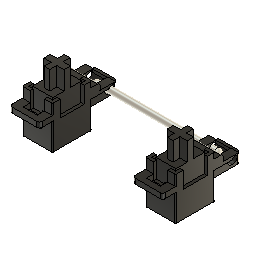
Choc v2 Stabilizer v8 (Autodesk Fusion 360 design; units mm, degrees)
Autodesk Fusion 360 part; units mm, degrees
note: some values were not read from the file. Chosen so that the rebuilt part matches the saved one: which bodies a step acts on; a side; which face or edge a step refers to.
ref_plane "WorkPlane1" through (0, 0, -5.4) normal (0, 0, 1) x (1, 0, 0)
ref_plane "Ext Bottom" through (0, 0, -2) normal (0, 0, 1) x (1, 0, 0)
ref_plane "WorkPlane3" through (0, 0, -0.2) normal (0, 0, 1) x (1, 0, 0)
sketch "Case Top" plane through (0, 0, 0) normal (0, 0, 1) x (1, 0, 0)
  line L0 (1.3, -2.05) -> (-1.3, -2.05)
  line L1 (-1.3, -2.05) -> (-1.3, 2.05)
  line L2 (-1.3, 2.05) -> (1.3, 2.05)
  line L3 (1.3, 2.05) -> (1.3, -2.05)
  line L4 (1.3, -2.05) -> (-1.3, 2.05) construction
  line L5 (-1.3, -2.05) -> (1.3, 2.05) construction
  line L6 (2.9, -3.8) -> (-2.9, -3.8)
  line L7 (-2.9, -3.8) -> (-2.9, 3.8)
  line L8 (-2.9, 3.8) -> (2.9, 3.8)
  line L9 (2.9, 3.8) -> (2.9, -3.8)
  line L10 (2.9, -3.8) -> (-2.9, 3.8) construction
  line L11 (-2.9, -3.8) -> (2.9, 3.8) construction
  line L12 (-2.9, -3.8) -> (2.9, -3.8)
  line L13 (2.9, -3.8) -> (2.9, -6.3)
  line L14 (2.9, -6.3) -> (-2.9, -6.3)
  line L15 (-2.9, -6.3) -> (-2.9, -3.8)
  line L16 (-2.9, 3.8) -> (2.9, 3.8)
  line L17 (2.9, 3.8) -> (2.9, 9.4)
  line L18 (2.9, 9.4) -> (-2.9, 9.4)
  line L19 (-2.9, 9.4) -> (-2.9, 3.8)
  line L20 (-2.9, 5.4) -> (2.9, 5.4)
  line L21 (-2.9, -2.3) -> (-2.3, -2.3)
  line L22 (-2.3, -2.3) -> (-2.3, -3.2)
  line L23 (-2.3, -3.2) -> (-1.4, -3.2)
  line L24 (-1.4, -3.2) -> (-1.4, -3.8)
  line L25 (0, 2.5) -> (0, 20)
  line L26 (2.9, -2.3) -> (2.3, -2.3)
  line L27 (2.3, -2.3) -> (2.3, -3.2)
  line L28 (2.3, -3.2) -> (1.4, -3.2)
  line L29 (1.4, -3.2) -> (1.4, -3.8)
  line L30 (20, 0) -> (2.5, 0)
  line L31 (-2.9, 2.3) -> (-2.3, 2.3)
  line L32 (-2.3, 2.3) -> (-2.3, 3.2)
  line L33 (-2.3, 3.2) -> (-1.4, 3.2)
  line L34 (-1.4, 3.2) -> (-1.4, 3.8)
  line L35 (1.4, 3.2) -> (1.4, 3.8)
  line L36 (2.3, 3.2) -> (1.4, 3.2)
  line L37 (2.3, 2.3) -> (2.3, 3.2)
  line L38 (2.9, 2.3) -> (2.3, 2.3)
  line L39 (-2.3, 2.3) -> (-2.3, -2.3)
  line L40 (2.3, -2.3) -> (2.3, 2.3)
  line L41 (-1.4, 3.2) -> (1.4, 3.2)
  line L42 (-1.4, -3.2) -> (1.4, -3.2)
  line L43 (2.15, 9.4) -> (2.15, 3.8)
  line L44 (-2.15, 9.4) -> (-2.15, 3.8)
  line L45 (-1, 9.4) -> (1, 9.4)
  line L46 (1, 9.4) -> (1, 9.9)
  line L47 (1, 9.9) -> (-1, 9.9)
  line L48 (-1, 9.9) -> (-1, 9.4)
  line L49 (-2.9, 8.4) -> (2.9, 8.4)
  line L50 (-0.95, -3.8) -> (0.95, -3.8)
  line L51 (0.95, -3.8) -> (0.95, -4.8)
  line L52 (0.95, -4.8) -> (-0.95, -4.8)
  line L53 (-0.95, -4.8) -> (-0.95, -3.8)
  line L54 (1.4, 8.4) -> (1.4, 3.8)
  line L55 (-1.4, 8.4) -> (-1.4, 3.8)
  line L56 (11.7972, 15.6555) -> (-12.0028, 15.6555)
  dimension "d3" = 2.6
  dimension "d4" = 4.1
  dimension "d5" = 7.6
  dimension "d6" = 5.8
  dimension "d7" = 2.5
  dimension "d8" = 5.6
  dimension "d9" = 4
  dimension "d10" = 1.5
  dimension "d11" = 1.5
  dimension "d12" = 0.6
  dimension "d13" = 0.6
  dimension "d14" = 4.3
  dimension "d16" = 2
  dimension "d17" = 0.5
  dimension "d26" = 4.6
  dimension "d36" = 1.9
  dimension "d37" = 1
  dimension "d49" = 2.8
  dimension "ParameterA" = 23.8
  constraint horizontal L0
  constraint perpendicular L0 L1
  constraint parallel L0 L2
  constraint parallel L1 L3
  constraint coincident L4 origin
  constraint coincident L5 origin
  constraint horizontal L6
  constraint perpendicular L6 L7
  constraint parallel L6 L8
  constraint parallel L7 L9
  constraint coincident L10 origin
  constraint coincident L11 origin
  constraint horizontal L12
  constraint vertical L13
  constraint horizontal L14
  constraint vertical L15
  constraint coincident L6.start L9.end
  constraint horizontal L16
  constraint vertical L17
  constraint horizontal L18
  constraint vertical L19
  constraint coincident L8.end L9.start
  constraint coincident L19 L20.start
  constraint coincident L17 L20.end
  constraint perpendicular L17 L20
  constraint coincident L7 L21.start
  constraint perpendicular L7 L21
  constraint perpendicular L21 L22
  constraint perpendicular L22 L23
  constraint coincident L12 L24.end
  constraint vertical L24
  constraint symmetric L21.start L25 L26.start
  constraint symmetric L21.end L25 L26.end
  constraint symmetric L22.end L25 L27.end
  constraint symmetric L23.end L25 L28.end
  constraint symmetric L24.end L25 L29.end
  constraint symmetric L21.start L30 L31.start
  constraint symmetric L21.end L30 L31.end
  constraint symmetric L22.end L30 L32.end
  constraint symmetric L23.end L30 L33.end
  constraint symmetric L24.end L30 L34.end
  constraint symmetric L26.start L30 L38.start
  constraint symmetric L26.end L30 L37.start
  constraint symmetric L27.end L30 L36.start
  constraint symmetric L28.end L30 L35.start
  constraint symmetric L29.end L30 L35.end
  constraint coincident L18 L43.start
  constraint coincident L16 L43.end
  constraint perpendicular L16 L43
  constraint symmetric L25 L43.start L44.start
  constraint symmetric L25 L43.end L44.end
  constraint horizontal L45
  constraint vertical L46
  constraint horizontal L47
  constraint vertical L48
  constraint coincident L18 L45.start
  constraint symmetric L25 L46 L48
  constraint coincident L19 L49.start
  constraint coincident L17 L49.end
  constraint perpendicular L17 L49
  constraint horizontal L50
  constraint vertical L51
  constraint horizontal L52
  constraint vertical L53
  constraint coincident L6 L50.start
  constraint symmetric L25 L51 L53
  constraint coincident L49 L54.start
  constraint coincident L16 L35.end
  constraint vertical L54
  constraint symmetric L25 L54.start L55.start
  constraint symmetric L25 L35.end L34.end
  constraint horizontal L56
  measures "d3" distance of L0.start L0.end
  measures "d4" distance of L0.start L2.end
  measures "d5" distance of L6.start L8.end
  measures "d6" distance of L6.start L6.end
  measures "d7" distance of L6.start L13.end
  measures "d8" distance of L8.end L17.end
  measures "d9" distance of L18 L20
  measures "d10" distance of L7 L24
  measures "d11" distance of L6 L21
  measures "d12" distance of L21.start L21.end
  measures "d13" distance of L23.end L24.end
  measures "d14" distance of L43 L44
  measures "d16" distance of L46.end L47.end
  measures "d17" distance of L45.end L46.end
  measures "d26" distance of L8 L49
  measures "d36" distance of L51.end L52.end
  measures "d37" distance of L50.end L51.end
  measures "d49" distance of L54 L55
  measures "ParameterA" distance of L56.start L56.end
extrude "Extrude1" add sketch "Case Top" against normal up to surface (5.2 mm away) from surface at -0.2 contours L0 L1 L2 L3 | L6 L9 L12 L26 L27 L28 L29 | L6 L12 L24 L29 L42 L50 | L9 L26 L38 L40 | L22 L23 L27 L28 L32 L33 L36 L37 L39 L40 L41 L42 | L6 L7 L12 L21 L22 L23 L24 | L8 L9 L16 L35 L36 L37 L38 | L7 L21 L31 L39 | L8 L16 L25 L35 L41 | L7 L8 L16 L31 L32 L33 L34 | L8 L16 L25 L34 L41 makes body 1
extrude "Extrude2" add sketch "Case Top" along normal blind 3.2 from surface at -0.2 contours L6 L9 L12 L26 L27 L28 L29 | L6 L7 L12 L21 L22 L23 L24 | L8 L9 L16 L35 L36 L37 L38 | L7 L8 L16 L31 L32 L33 L34 bodies 1
extrude "Extrude4" cut sketch "Case Top" against normal up to surface (5.4 mm away) contours L0 L1 L2 L3 bodies 1
extrude "Extrude3" cut sketch "Case Top" against normal up to surface (4.8 mm away) contours L22 L23 L27 L28 L32 L33 L36 L37 L39 L40 L41 L42 bodies 1
extrude "Extrude5" add sketch "Case Top" along normal blind 0.6 separate body contours L8 L16 L17 L20 L43 | L8 L16 L20 L43 L54 | L17 L20 L43 L49 | L8 L16 L20 L25 L54 | L20 L43 L49 L54 | L8 L16 L19 L20 L44 | L8 L16 L20 L25 L55 | L20 L25 L49 L54 | L8 L16 L20 L44 L55 | L19 L20 L44 L49 | L20 L25 L49 L55 | L20 L44 L49 L55 makes body 2
extrude "Extrude6" add sketch "Case Top" along normal blind 1.9 contours L8 L16 L17 L20 L43 | L8 L16 L20 L43 L54 | L8 L16 L20 L25 L54 | L8 L16 L19 L20 L44 | L8 L16 L20 L25 L55 | L8 L16 L20 L44 L55 bodies 1 2
extrude "Extrude7" add sketch "Case Top" against normal up to surface (2 mm away) contours L8 L16 L20 L43 L54 | L8 L16 L20 L25 L54 | L20 L43 L49 L54 | L8 L16 L20 L25 L55 | L20 L25 L49 L54 | L18 L25 L43 L45 L49 | L8 L16 L20 L44 L55 | L20 L25 L49 L55 | L20 L44 L49 L55 | L18 L25 L44 L45 L49 bodies 1
extrude "Extrude8" add sketch "Case Top" against normal blind 1 from surface at -1 contours L18 L25 L45 L46 L47 | L18 L25 L45 L47 L48 bodies 1
extrude "Extrude9" add sketch "Case Top" along normal blind 1 contours L6 L12 L13 L14 L15 L51 L52 L53 bodies 1
extrude "Extrude10" add sketch "Case Top" against normal blind 1.5 from surface at -0.5 contours L6 L12 L50 L51 L52 L53 bodies 1
extrude "Extrude11" cut sketch "Case Top" along normal up to surface (0.6 mm away) and the other way blind 1.4 contours L8 L16 L20 L25 L54 | L8 L16 L20 L25 L55 | L20 L25 L49 L54 | L20 L25 L49 L55 bodies 1
fillet "Fillet1" radius 0.2 16 edges at (-2.9, 3.8, -2.7) (0, 3.8, -5.4) (2.9, 3.8, -2.7) (-2.9, 3.8, 2.45) (-2.9, -3.8, 2) (-2.9, -3.8, -2.7) (-2.9, 0, -5.4) (2.9, 0, -5.4) (0, -3.8, -5.4) (2.9, -3.8, -2.7) (2.9, -3.8, 2) (2.9, 3.8, 2.45) (1.3, -2.05, -5.1) (1.3, 2.05, -5.1) (-1.3, 2.05, -5.1) (-1.3, -2.05, -5.1) on bodies 1
fillet "Fillet2" radius 0.5 5 edges at (0, 5.4, 1.9) (-2.15, 9.4, -1) (2.15, 9.4, -1) (-2.9, -6.3, 0.5) (2.9, -6.3, 0.5) on bodies 1
chamfer "Chamfer1" distance 0.7 angle 45 2 edges at (0, -4.8, -0.5) (0, -4.8, -2) on bodies 1
chamfer "Chamfer2" distance 0.5 angle 45 1 edges at (0, 9.9, -2) on bodies 1
move_face "OffsetFaces1" offset -0.4 3 faces at (0.3167, -4.8, 0.3333) (0.95, -4.1333, 0.3333) (-0.95, -4.4667, 0.3333) on bodies 1
sketch "Case Side2" plane through (-2.15, 0, 0) normal (-1, 0, 0) x (0, -1, 0)
  line L0 (-8.4, -1.4) -> (-3.8, -1.4)
  arc A0 (-8.8655, -0.5741) -> (-8.4, -1.4) centre (-7.9, -0.5741) ccw
  line L1 (-8.8655, -0.5741) -> (-8.8655, 0.3914)
  circle A1 centre (-7.9, -0.8) radius 0.6
  arc A2 (-8.4, -1.4) -> (-7.9, 0.3914) centre (-7.9, -0.5741) ccw
  line L2 (-8.4, 0) -> (-8.4, 0.6)
  line L3 (-7.9, 0.3914) -> (-8.8655, 0.3914)
  line L4 (-7.9, -1.1252) -> (-7.9, 0.2054) construction
  dimension "d55" = 1.2
  dimension "WireYAdjust" = 0.5
  constraint coincident L0.start A0.end
  constraint perpendicular L0 L1
  constraint tangent A0 L1
  constraint tangent L0 A1
  constraint tangent A0 A2
  constraint horizontal L3
  constraint coincident L1.end L3.end
  constraint vertical L4
  constraint coincident A1.centre L4
  constraint coincident A0.centre L4
  constraint tangent A2 L3
  measures "d55" diameter of A1
  measures "WireYAdjust" distance of A1.centre L2
extrude "Extrude12" cut sketch "Case Side2" along normal up to surface (-5.05 mm away) and the other way up to surface (-0.75 mm away) contours A1 | L0 A0 L1 A2 L3 | L0 A2 bodies 1
sketch "Stem Top" plane through (0, 0, -0.2) normal (0, 0, 1) x (1, 0, 0)
  line L0 (-1.95, 2.8) -> (1.95, 2.8)
  line L1 (1.95, 2.8) -> (1.95, -2.8)
  line L2 (1.95, -2.8) -> (-1.95, -2.8)
  line L3 (-1.95, -2.8) -> (-1.95, 2.8)
  line L4 (-1.95, 2.8) -> (1.95, -2.8) construction
  line L5 (1.95, 2.8) -> (-1.95, -2.8) construction
  line L6 (-0.55, -0.615) -> (-1.95, -0.615)
  line L7 (-0.55, -0.615) -> (-0.55, -1.95)
  line L8 (20, 0) -> (2.5, 0)
  line L9 (-0.55, 0.615) -> (-1.95, 0.615)
  line L10 (-0.55, 0.615) -> (-0.55, 1.95)
  line L11 (0, 2.5) -> (0, 20)
  line L12 (0.55, -0.615) -> (1.95, -0.615)
  line L13 (0.55, -0.615) -> (0.55, -1.95)
  line L14 (0.55, 0.615) -> (0.55, 1.95)
  line L15 (0.55, 0.615) -> (1.95, 0.615)
  line L16 (0.55, -1.95) -> (-0.55, -1.95)
  line L17 (0.55, 1.95) -> (-0.55, 1.95)
  dimension "d60" = 3.9
  dimension "d61" = 5.6
  dimension "d62" = 1.23
  dimension "d63" = 1.1
  dimension "d64" = 3.9
  constraint horizontal L0
  constraint perpendicular L0 L1
  constraint parallel L0 L2
  constraint parallel L1 L3
  constraint coincident L4 origin
  constraint coincident L5 origin
  constraint coincident L3 L6.end
  constraint perpendicular L3 L6
  constraint perpendicular L6 L7
  constraint symmetric L6.start L8 L9.start
  constraint symmetric L6.end L8 L9.end
  constraint symmetric L7.end L8 L10.end
  constraint symmetric L6.start L11 L12.start
  constraint symmetric L6.end L11 L12.end
  constraint symmetric L7.end L11 L13.end
  constraint symmetric L9.start L11 L14.start
  constraint symmetric L9.end L11 L15.end
  constraint symmetric L10.end L11 L14.end
  measures "d60" distance of L0.start L0.end
  measures "d61" distance of L0.start L2.end
  measures "d62" distance of L6 L9
  measures "d63" distance of L7 L13
  measures "d64" distance of L16 L17
extrude "Extrude13" add sketch "Stem Top" along normal blind 3.6 separate body contours L1 L3 L6 L7 L9 L10 L12 L13 L14 L15 L16 L17 makes body 3
extrude "Extrude14" add sketch "Stem Top" against normal blind 4.5 bodies 3
move_body "Move2" bodies 3 to x (1, 0, 0) y (0, 1, 0) z (0, 0, 1) at (0, 0, 3.2)
sketch "Fill Hole Top" plane through (0, 0, 0) normal (0, 0, 1) x (1, 0, 0)
  line L0 (3, -4.5) -> (-3, -4.5)
  line L1 (-3, -4.5) -> (-3, 9.4)
  line L2 (-3, 9.4) -> (3, 9.4)
  line L3 (3, 9.4) -> (3, -4.5)
  line L4 (3, -4.5) -> (-3, 9.4) construction
  line L5 (-3, -4.5) -> (3, 9.4) construction
  line L6 (0, 1.75) -> (0, 22.5)
  line L7 (-4, -5.5) -> (-4, 10.4)
  line L8 (-4, 10.4) -> (4, 10.4)
  line L9 (4, 10.4) -> (4, -5.5)
  line L10 (4, -5.5) -> (-4, -5.5)
  line L11 (2.25, 9.4) -> (2.25, 3.9)
  line L12 (2.25, 3.9) -> (3, 3.9)
  line L13 (2.15, 9.4) -> (2.15, 3.8)
  line L14 (-2.9, 3.8) -> (2.9, 3.8)
  line L15 (0, 2.5) -> (0, 20)
  line L16 (-2.25, 3.9) -> (-3, 3.9)
  line L17 (-2.25, 9.4) -> (-2.25, 3.9)
  line L18 (-2.4, -6.3) -> (2.4, -6.3)
  arc A0 (-2.9, -5.8) -> (-2.4, -6.3) centre (-2.4, -5.8) ccw
  line L19 (-2.9, -3.6) -> (-2.9, -5.8)
  arc A1 (2.4, -6.3) -> (2.9, -5.8) centre (2.4, -5.8) ccw
  line L20 (2.9, -5.8) -> (2.9, -3.6)
  line L21 (-3, -3.6) -> (-3, -5.8)
  arc A2 (-3, -5.8) -> (-2.4, -6.4) centre (-2.4, -5.8) ccw
  line L22 (-2.4, -6.4) -> (2.4, -6.4)
  arc A3 (2.4, -6.4) -> (3, -5.8) centre (2.4, -5.8) ccw
  line L23 (3, -5.8) -> (3, -3.6)
  line L24 (-2.25, 3.9) -> (2.25, 3.9)
  point P0 (0, 2.45)
  point P1 (-2.15, 9.4)
  dimension "d72" = 6
  dimension "d74" = -1
  dimension "d76" = 0.1
  dimension "d77" = 0.1
  dimension "d78" = 8.3
  dimension "d85" = 0.1
  constraint horizontal L0
  constraint perpendicular L0 L1
  constraint parallel L0 L2
  constraint parallel L1 L3
  constraint coincident L4 P0
  constraint coincident L5 P0
  constraint coincident P0 L6
  constraint coincident L2 P1
  constraint coincident L2 L11.start
  constraint perpendicular L2 L11
  constraint coincident L3 L12.end
  constraint perpendicular L3 L12
  constraint symmetric L11.start L15 L17.start
  constraint symmetric L11.end L15 L16.start
  constraint symmetric L12.end L15 L16.end
  measures "d72" distance of L0.start L0.end
  measures "d76" distance of L11 L13
  measures "d77" distance of L12 L14
  measures "d78" distance of L0 L14
extrude "Extrude15" add sketch "Fill Hole Top" against normal blind 5.5 separate body contours L0 L10 L20 L23 | L0 L1 L3 L6 L12 L13 L14 L15 L16 L21 L23 L24 | L2 L3 L6 L8 L9 L10 L15 L23 | L0 L10 L19 L20 | L0 L10 L19 L21 | L2 L3 L11 L12 | L1 L2 L6 L7 L8 L10 L15 L21 | L2 L11 L13 L24 | L2 L6 L13 L15 L24 | L6 L13 L14 L15 L24 | L1 L2 L16 L17 | L2 L6 L15 L17 L24 makes body 4
extrude "Extrude16" add sketch "Fill Hole Top" against normal up to surface (2.1 mm away) separate body contours L0 L1 L3 L6 L12 L13 L14 L15 L16 L21 L23 L24 | L2 L11 L13 L24 | L2 L6 L13 L15 L24 | L6 L13 L14 L15 L24 | L2 L6 L15 L17 L24 makes body 5
sketch "Jaw 1" plane through (0, 9.4, 0) normal (0, 1, 0) x (-1, 0, 0)
  line L0 (-2.25, -2.1) -> (2.25, -2.1)
  line L1 (2.25, -2.1) -> (2.25, 0)
  line L2 (2.25, 0) -> (-2.25, 0)
  line L3 (-2.25, 0) -> (-2.25, -2.1)
  line L4 (-2.25, -1) -> (2.25, -1)
  point P0 (-1, -1)
  constraint coincident L3 L4.start
  constraint coincident L1 L4.end
  constraint perpendicular L1 L4
  constraint coincident L4 P0
extrude "Extrude17" add sketch "Jaw 1" along normal blind 1 contours L0 L1 L3 L4 bodies 5
sketch "Jaw 2" plane through (0, -4.5, 0) normal (0, -1, 0) x (1, 0, 0)
  line L0 (-3, -2.1) -> (3, -2.1)
  line L1 (3, -2.1) -> (3, 0)
  line L2 (3, 0) -> (-3, 0)
  line L3 (-3, 0) -> (-3, -2.1)
  line L4 (-1.25, -2.1) -> (1.25, -2.1)
  line L5 (1.25, -2.1) -> (1.25, -1)
  line L6 (1.25, -1) -> (-1.25, -1)
  line L7 (-1.25, -1) -> (-1.25, -2.1)
  line L8 (-2.4, 0) -> (2.4, 0)
  line L9 (0, 1.75) -> (0, 22.5)
  dimension "d86" = 1
  dimension "d87" = 2.5
  constraint horizontal L4
  constraint vertical L5
  constraint horizontal L6
  constraint vertical L7
  constraint coincident L0 L4.start
  constraint symmetric L5 L7 L9
  measures "d86" distance of L6 L8
  measures "d87" distance of L5.end L6.end
extrude "Extrude18" add sketch "Jaw 2" along normal blind 0.5 contours L0 L4 L5 L6 L7 bodies 5
extrude "Extrude19" add sketch "Fill Hole Top" against normal up to surface (5.5 mm away) contours L0 L1 L3 L6 L12 L13 L14 L15 L16 L21 L23 L24 | L6 L13 L14 L15 L24 bodies 5
extrude "Extrude20" add sketch "Fill Hole Top" along normal blind 8 contours L0 L10 L20 L23 | L0 L1 L3 L6 L12 L13 L14 L15 L16 L21 L23 L24 | L0 L10 L19 L20 | L10 L18 A0 L19 A1 L20 L21 A2 L22 A3 L23 | L0 L10 L19 L21 | L10 L18 A0 L19 A1 L20 | L2 L3 L11 L12 | L2 L11 L13 L24 | L2 L6 L13 L15 L24 | L6 L13 L14 L15 L24 | L1 L2 L16 L17 | L2 L6 L15 L17 L24 bodies 5
copy_body "CopyPasteBodies1" bodies 1 makes body 6
extrude "Extrude23" add sketch "Fill Hole Top" against normal blind 1 separate body contours L0 L10 L19 L20 | L2 L3 L11 L12 | L1 L2 L16 L17 makes body 7 at (2.25, 7.5667, -0.3333) makes body 8 at (-3, 5.7333, -0.3333) makes body 9 at (0.9667, -5.5, -0.3333)
move_face "OffsetFaces3" offset -2 2 faces at (-2.75, 9.4, -0.3333) (2.5, 9.4, -0.3333) on bodies 7 8
ref_plane "WorkPlane4" through (0, 0, -0.8) normal (0, 0, 1) x (1, 0, 0)
sketch "Wire" plane through (0, 0, -0.8) normal (0, 0, 1) x (1, 0, 0)
  line L0 (11.1, 7.9) -> (-11.1, 7.9)
  line L1 (0, 1.75) -> (0, 22.5)
  line L2 (12.1, 6.9) -> (12.1, -2.7)
  line L3 (0, 2.5) -> (0, 20)
  line L4 (-12.1, 6.9) -> (-12.1, -2.7)
  arc A0 (12.1, 6.9) -> (11.1, 7.9) centre (11.1, 6.9) ccw
  arc A1 (-11.1, 7.9) -> (-12.1, 6.9) centre (-11.1, 6.9) ccw
  point P0 (-2.15, 7.9)
  point P1 (12.1, 7.9)
  point P2 (-12.1, 7.9)
  dimension "d96" = 24.2
  dimension "d97" = 10.6
  dimension "d98" = 1
  constraint horizontal L0
  constraint symmetric P1 P2 L1
  constraint coincident P0 L0
  constraint perpendicular L0 L2
  constraint symmetric L2.end L3 L4.end
  constraint coincident P1 L0
  constraint coincident P1 L2
  constraint tangent L0 A0
  constraint tangent L2 A0
  constraint coincident P2 L0
  constraint tangent L4 A1
  constraint tangent L0 A1
  constraint equal A0 A1
  constraint vertical L4
  measures "d96" distance of P1 P2
  measures "d97" distance of P1 L2.end
  measures "d98" radius of A0
pipe "Pipe1" add diameter 1.2 path "Wire" along L4 A1 L0 A0 L2 separate body makes body 10
copy_body "CopyPasteBodies2" bodies 10 makes body 11
pipe "Pipe2" add diameter 1.6 path "Wire" along L4 A1 L0 A0 L2 separate body makes body 12
sketch "Wire Insert Hole" plane through (0, 0, -0.8) normal (0, 0, 1) x (1, 0, 0)
  line L0 (11.3, 6.9) -> (11.3, -2.7)
  line L1 (11.3, -2.7) -> (12.9, -2.7)
  line L2 (12.9, -2.7) -> (12.9, 6.9)
  arc A0 (12.9, 6.9) -> (11.1, 8.7) centre (11.1, 6.9) ccw
  line L3 (11.1, 8.7) -> (-11.1, 8.7)
  arc A1 (-11.1, 8.7) -> (-12.9, 6.9) centre (-11.1, 6.9) ccw
  line L4 (-12.9, 6.9) -> (-12.9, -2.7)
  line L5 (-12.9, -2.7) -> (-11.3, -2.7)
  line L6 (-11.3, -2.7) -> (-11.3, 6.9)
  arc A2 (-11.3, 6.9) -> (-11.1, 7.1) centre (-11.1, 6.9) cw
  line L7 (-11.1, 7.1) -> (11.1, 7.1)
  arc A3 (11.1, 7.1) -> (11.3, 6.9) centre (11.1, 6.9) cw
extrude "Extrude21" add sketch "Wire Insert Hole" along normal blind 8 separate body makes body 13
combine "Combine1" operation add target body 12 tool bodies 13
move_body "Move1" bodies 1 3 7 8 9 4 5 6 to x (1, 0, 0) y (0, 1, 0) z (0, 0, 1) at (11.9, 0, 0)
combine "Combine5" operation cut target body 8 tool bodies 12 keep tools
mirror "Mirror1" about plane through (0, 0, 0) normal (1, 0, 0) of bodies 1 3 7 8 9 4 5 6 makes body 14 at (-9, 0.7667, -3.5333) makes body 15 at (-12.55, -0.9333, -1.5) makes body 16 at (-11.9, -0.2, 0) makes body 17 at (-8.9, 2.5, 5.3333) makes body 18 at (-9, 0.7667, -3.5333) makes body 19 at (-14.9, 6.2333, -0.3333) makes body 20 at (-8.9, 4.9667, -0.6) makes body 21 at (-12.8667, -5.1667, -1)
copy_body "CopyPasteBodies3" bodies 12 makes body 22
combine "Combine2" operation add target body 22 tool bodies 5 17 keep tools
combine "Combine3" operation add target body 11 tool bodies 18 6
move_body "Move3" bodies 1 3 7 8 9 4 5 10 12 14 15 19 20 21 16 17 11 22 to x (1, 0, 0) y (0, 1, 0) z (0, 0, 1) at (0, 0.3, 0)
hidden bodies 11 22 4 5 7 8 9 12 16 17 19 20 21
equation "d96 = ParameterA + 0.4 mm"
named bodies: "Case", "Stem", "Fill", "Hole", "MEV", "Placeholder", "MEV (1)", "Wire Hole", "Wire Insert Hole", "MF", "MF (2)", "MF (1)", "Case (1)", "Stem (1)", "Fill (1)", "Hole (1)", "MF (3)", "MF (2) (1)", "MF (1) (1)", "Territory"
